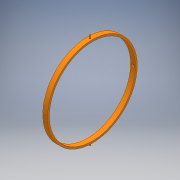
# Autodesk Inventor part: Inner Ring
Saved by Autodesk Inventor 2018 (Build 220112000, 112)
## iProperties
Created: 2018-03-06
Part Number: Inner Ring
Material: Generic
Document SubType Name: Modeling
Designer: sterl
Density: 1 g/cm^3
Appearance: Orange
Author: sterl
Autodesk Inventor part; units mm, degrees
sketch "Sketch1" plane through (0, 0, 0) normal (1, 0, 0) x (0, 1, 0)
  circle A0 centre (0, 0) radius 90
  circle A1 centre (0, 0) radius 94
  dimension "d0" = 180
  dimension "d1" = 188
  constraints: 2 centre point, 2 coincident
  measures "d0" diameter of A0
  measures "d1" diameter of A1
extrude "Extrusion1" add sketch "Sketch1" along normal blind 10
ref_plane "Work Plane1" through (0, 94, 0) normal (0, 1, 0) x (-1, 0, 0)
sketch "Sketch2" plane through (0, 94, 0) normal (0, 1, 0) x (-1, 0, 0)
  line L0 (-10, 94) -> (-10, -94) projected
  line L1 (0, -94) -> (0, 94) projected
  line L2 (0, 0) -> (-10, 0)
  circle A0 centre (-5, 0) radius 3
  circle A1 centre (-5, 0) radius 1.5
  dimension "d4" = 6
  dimension "d5" = 3
  constraints: 2 centre point, 2 end point, 2 midpoint, 1 coincident
  measures "d4" diameter of A0
  measures "d5" diameter of A1
extrude "Extrusion2" cut sketch "Sketch2" against normal blind 230 contours A1 L2 | L2 A1
ref_plane "Work Plane2" through (0, -90, 0) normal (0, 1, 0) x (-1, 0, 0)
sketch "Sketch3" plane through (0, -90, 0) normal (0, 1, 0) x (-1, 0, 0)
  line L0 (-3.5, 0) -> (-6.5, 0)
  circle A0 centre (-5, 0) radius 3
  point P0 (0, 0)
  dimension "d8" = 6
  constraints: 2 end point, 1 centre point, 1 horizontal, 1 midpoint, 3 other
  measures "d8" diameter of A0
extrude "Extrusion3" cut sketch "Sketch3" along normal mid plane 5
ref_plane "Work Plane3" through (0, 90, 0) normal (0, 1, 0) x (-1, 0, 0)
sketch "Sketch4" plane through (0, 90, 0) normal (0, 1, 0) x (-1, 0, 0)
  spline S0 degree 7 poles (-3.5, 0) (-3.5, 0.2132) (-3.5353, 0.4207) (-3.6027, 0.6159) (-3.6973, 0.7932) (-3.8134, 0.9484) (-3.9438, 1.0791) (-4.1987, 1.2768) (-4.3241, 1.3521) (-4.4547, 1.4117) (-4.5888, 1.456) (-4.7252, 1.4853) (-4.8627, 1.5) (-5.1374, 1.5) (-5.2748, 1.4853) (-5.4112, 1.4559) (-5.5453, 1.4117) (-5.6759, 1.3521) (-5.8013, 1.2768) (-6.0307, 1.0989) (-6.1365, 0.9972) (-6.2337, 0.8802) (-6.3191, 0.7485) (-6.3894, 0.6034) (-6.4418, 0.4468) (-6.5071, 0.1046) (-6.5164, -0.0779) (-6.4994, -0.2608) (-6.4568, -0.4377) (-6.3913, -0.6029) (-6.3079, -0.7518) (-6.1505, -0.9685) (-6.0817, -1.048) (-6.0081, -1.1201) (-5.9305, -1.1849) (-5.8497, -1.2425) (-5.7664, -1.293) (-5.5883, -1.3837) (-5.4932, -1.4227) (-5.3963, -1.4537) (-5.2981, -1.4769) (-5.199, -1.4923) (-5.0995, -1.5) (-4.8626, -1.5) (-4.7252, -1.4853) (-4.5888, -1.4559) (-4.4547, -1.4117) (-4.3241, -1.3521) (-4.1987, -1.2768) (-3.9439, -1.0791) (-3.8134, -0.9485) (-3.6973, -0.7932) (-3.6026, -0.6159) (-3.5353, -0.4206) (-3.5, -0.2131) (-3.5, 0) knots 0 0 0 0 0 0 0 0 0.133551 0.133551 0.133551 0.133551 0.133551 0.133551 0.248756 0.248756 0.248756 0.248756 0.248756 0.248756 0.36403 0.36403 0.36403 0.36403 0.36403 0.36403 0.472701 0.472701 0.472701 0.472701 0.472701 0.472701 0.588434 0.588434 0.588434 0.588434 0.588434 0.588434 0.665803 0.665803 0.665803 0.665803 0.665803 0.665803 0.749751 0.749751 0.749751 0.749751 0.749751 0.749751 0.865692 0.865692 0.865692 0.865692 0.865692 0.865692 1 1 1 1 1 1 1 1 projected
  line L0 (-6.5, 0) -> (-3.5, 0)
  circle A0 centre (-5, 0) radius 3
  point P0 (0, 0)
  dimension "d12" = 6
  constraints: 2 end point, 1 centre point, 1 horizontal, 1 midpoint, 3 other
  measures "d12" diameter of A0
extrude "Extrusion4" cut sketch "Sketch4" along normal mid plane 5
ref_plane "Work Plane4" through (0, 0, 94) normal (0, 0, 1) x (1, 0, 0)
sketch "Sketch5" plane through (0, 0, 94) normal (0, 0, 1) x (1, 0, 0)
  line L0 (10, -94) -> (10, 94) projected
  line L1 (0, 94) -> (0, -94) projected
  line L2 (0, 0) -> (10, 0)
  line L3 (10, 90) -> (10, -90) projected
  circle A0 centre (5, 0) radius 1.5
  dimension "d15" = 3
  constraints: 2 end point, 2 midpoint, 1 centre point
  measures "d15" diameter of A0
extrude "Extrusion5" add sketch "Sketch5" along normal mid plane 12
mirror "Mirror1" about plane through (0, 0, 0) normal (0, 0, 1) of "Extrusion5"
sketch "Sketch6" plane through (10, 0, 0) normal (1, 0, 0) x (0, 0, -1)
  circle A0 centre (0, 0) radius 90 projected
extrude "Extrusion6" cut sketch "Sketch6" against normal blind 8
body "Solid1"
